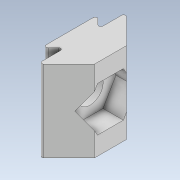
# Autodesk Inventor part: nut
Saved by Autodesk Inventor 2020 (Build 240168000, 168)
## iProperties
Created: 2020-08-24
Part Number: nut
Material: Generic
Document SubType Name: Modeling
Designer: Admin
Density: 1 g/cm^3
Appearance: Default
Author: Admin
Autodesk Inventor part; units mm, degrees
ref_plane "YZ Plane" through (0, 0, 0) normal (1, 0, 0) x (0, 1, 0)
ref_plane "XZ Plane" through (0, 0, 0) normal (0, 1, 0) x (-1, 0, 0)
ref_plane "XY Plane" through (0, 0, 0) normal (0, 0, 1) x (1, 0, 0)
sketch "Sketch1" plane through (0, 0, 0) normal (0, 1, 0) x (-1, 0, 0)
  line L0 (0, 0) -> (3.5355, 3.5355)
  line L1 (3.5355, 3.5355) -> (3.5355, 0.0355)
  line L2 (3.5355, 0.0355) -> (5.0355, 1.5355)
  line L3 (5.0355, 1.5355) -> (5.0355, -5.4645)
  line L4 (5.0355, -5.4645) -> (3.5355, -3.9645)
  line L5 (3.5355, -3.9645) -> (3.5355, -7.4645)
  line L6 (3.5355, -7.4645) -> (0, -3.929)
  line L7 (0, -3.929) -> (0, 0)
  dimension "d0" = 3.929
  dimension "d1" = 5
  dimension "d2" = 5
  dimension "d3" = 3.5
  dimension "d4" = 3.5
  dimension "d5" = 135
  dimension "d6" = 45
  dimension "d7" = 1.5
  constraints: 16 end point, 2 parallel, 2 point on line, 1 perpendicular, 1 vertical
  measures "d0" distance of L6.end L0.start
  measures "d1" distance of L0.start L0.end
  measures "d2" distance of L5.end L6.end
  measures "d3" distance of L0.end L1.end
  measures "d4" distance of L4.end L5.end
  measures "d5" angle of L7 L0
  measures "d6" angle of L1 L2
  measures "d7" distance between parallel lines of L1 L3
extrude "Extrusion1" add sketch "Sketch1" along normal blind 10
fillet "Fillet1" radius 0.25 6 edges at (-3.5355, 5, -3.9645) (-3.5355, 5, -7.4645) (-5.0355, 5, -5.4645) (-3.5355, 5, 3.5355) (-3.5355, 5, 0.0355) (-5.0355, 5, 1.5355)
sketch "Sketch2" plane through (0, 0, 0) normal (1, 0, 0) x (0, 0, -1)
  line L0 (0.3768, 7.75) -> (3.5522, 7.75)
  line L1 (3.5522, 7.75) -> (5.1399, 5)
  line L2 (5.1399, 5) -> (3.5522, 2.25)
  line L3 (3.5522, 2.25) -> (0.3768, 2.25)
  line L4 (0.3768, 2.25) -> (-1.2109, 5)
  line L5 (-1.2109, 5) -> (0.3768, 7.75)
  line L6 (3.929, 0) -> (3.929, 10) projected
  line L7 (0, 10) -> (3.929, 10) projected
  point P0 (0, 0)
  point P1 (1.9645, 5)
  dimension "d11" = 5.5
  dimension "d12" = 1.9645
  dimension "d13" = 5
  constraints: 12 end point, 1 horizontal, 13 other
  measures "d11" distance between parallel lines of L5 L2
  measures "d12" distance from line of L6 point (1.965, 5)
  measures "d13" distance from line of L7 point (1.965, 5)
extrude "Extrusion2" cut sketch "Sketch2" against normal blind 2.5
sketch "Sketch3" plane through (-2.5, 0, 0) normal (1, 0, 0) x (0, 0, -1)
  circle A0 centre (1.9645, 5) radius 1.6
  line L0 (3.929, 0) -> (3.929, 2.9026) projected
  line L1 (0, 10) -> (3.929, 10) projected
  point P0 (0, 0)
  dimension "d16" = 3.2
  dimension "d17" = 1.9645
  dimension "d18" = 5
  constraints: 1 centre point
  measures "d16" diameter of A0
  measures "d17" distance from line of L0 A0.centre
  measures "d18" distance from line of L1 A0.centre
extrude "Extrusion3" cut sketch "Sketch3" against normal through all
body "Solid1"
